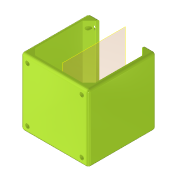
# Autodesk Inventor part: 55_spiralxy_slidemount_MGN9_Nema17_Body
Saved by Autodesk Inventor 2022 (Build 260153000, 153)
## iProperties
Created: 2019-07-01
Part Number: 55_spiralxy_slidemount_MGN9_Nema17_Body
Material: Generic
Document SubType Name: Modeling
Designer: diederichbenedict
Density: 1 g/cm^3
Appearance: IPHT_Grün
Author: diederichbenedict
Autodesk Inventor part; units mm, degrees
ref_plane "YZ Plane" through (0, 0, 0) normal (1, 0, 0) x (0, 1, 0)
ref_plane "XZ Plane" through (0, 0, 0) normal (0, 1, 0) x (-1, 0, 0)
ref_plane "XY Plane" through (0, 0, 0) normal (0, 0, 1) x (1, 0, 0)
sketch "Sketch1" plane through (0, 0, 0) normal (0, 0, 1) x (1, 0, 0)
  line L0 (-24.9, 24.9) -> (24.9, 24.9)
  line L1 (24.9, 24.9) -> (24.9, -24.9)
  line L2 (24.9, -24.9) -> (-24.9, -24.9)
  line L3 (-24.9, -24.9) -> (-24.9, 24.9)
  line L4 (-24.9, 24.9) -> (24.9, -24.9) construction
  line L5 (24.9, 24.9) -> (-24.9, -24.9) construction
  line L6 (17.05, 17.05) -> (-17.05, 17.05)
  line L7 (-17.05, 17.05) -> (-17.05, -17.05)
  line L8 (-17.05, -17.05) -> (17.05, -17.05)
  line L9 (17.05, -17.05) -> (17.05, 17.05)
  point P0 (0, 0)
  dimension "d0" = 49.8
  dimension "d1" = 49.8
  dimension "d2" = 7.85
  constraints: 20 end point, 4 parallel, 2 midpoint, 2 perpendicular, 1 horizontal, 3 other
  measures "d0" distance of L1.end L2.end
  measures "d1" distance of L0.end L1.end
  measures "d2" distance between parallel lines of L0 L6
extrude "Extrusion1" add sketch "Sketch1" along normal blind 7.7 contours L0 L1 L2 L3 | L9 L8 L7 L6
sketch "Sketch2" plane through (0, 0, 7.7) normal (0, 0, 1) x (1, 0, 0)
  line L0 (24.9, 24.9) -> (-24.9, 24.9) projected
  line L1 (-24.9, 24.9) -> (-24.9, -24.9) projected
  line L2 (-24.9, -24.9) -> (24.9, -24.9) projected
  line L3 (24.9, -24.9) -> (24.9, 24.9) projected
  line L4 (17.05, -17.05) -> (24.9, -17.05)
  line L5 (24.9, -17.05) -> (24.9, -24.9)
  line L6 (24.9, -24.9) -> (17.05, -24.9)
  line L7 (17.05, -24.9) -> (17.05, -17.05)
  line L8 (17.05, 17.05) -> (-17.05, 17.05) projected
  line L9 (24.9, 24.9) -> (17.05, 24.9)
  line L10 (17.05, 24.9) -> (17.05, 17.05)
  line L11 (17.05, 17.05) -> (24.9, 17.05)
  line L12 (24.9, 17.05) -> (24.9, 24.9)
  line L13 (-24.9, -24.9) -> (-17.05, -24.9)
  line L14 (-17.05, -24.9) -> (-17.05, -17.05)
  line L15 (-17.05, -17.05) -> (-24.9, -17.05)
  line L16 (-24.9, -17.05) -> (-24.9, -24.9)
  line L17 (-24.9, 24.9) -> (-17.05, 24.9)
  line L18 (-17.05, 24.9) -> (-17.05, 17.05)
  line L19 (-17.05, 17.05) -> (-24.9, 17.05)
  line L20 (-24.9, 17.05) -> (-24.9, 24.9)
  point P0 (0, 0)
  constraints: 32 end point, 8 parallel, 4 horizontal, 4 perpendicular
extrude "Extrusion2" add sketch "Sketch2" along normal blind 34.4
sketch "Sketch3" plane through (0, 0, 0) normal (0, 0, -1) x (-1, 0, 0)
  line L0 (24.9, -24.9) -> (24.9, 24.9) construction
  line L1 (24.9, 24.9) -> (-24.9, 24.9) construction
  line L2 (-24.9, -24.9) -> (24.9, -24.9) construction
  line L3 (-24.9, 24.9) -> (-24.9, -24.9) construction
  point P0 (20, 20)
  point P1 (20, -20)
  point P2 (-20, -20)
  point P3 (-20, 20)
  dimension "d_1" = 4.9
  dimension "d96" = 4.9
  dimension "d97" = 4.9
  dimension "d98" = 4.9
  dimension "d99" = 4.9
  dimension "d100" = 4.9
  dimension "d101" = 4.9
  dimension "d102" = 4.9
  measures "d_1" distance from line of L1 point (20, 20)
  measures "d96" distance from line of point (20, 20) L0
  measures "d97" distance from line of point (20, -20) L0
  measures "d98" distance from line of point (20, -20) L2
  measures "d99" distance from line of point (-20, -20) L2
  measures "d100" distance from line of point (-20, -20) L3
  measures "d101" distance from line of point (-20, 20) L3
  measures "d102" distance from line of point (-20, 20) L1
hole "Hole1" at (-20, 20, 0) at (-20, -20, 0) at (20, -20, 0) at (20, 20, 0) direction (0, 0, 1) diameter 2.8 end through all counterbore diameter 5.5 counterbore depth 3.1
fillet "Fillet1" radius 2 8 edges at (24.9, 24.9, 21.05) (24.9, -24.9, 21.05) (-24.9, -24.9, 21.05) (-24.9, 24.9, 21.05) (-24.9, 0, 0) (0, -24.9, 0) (24.9, 0, 0) (0, 24.9, 0)
sketch "Sketch9" plane through (0, 0, 42.1) normal (0, 0, 1) x (1, 0, 0)
  arc A0 (19.486, 18.6978) -> (18.6978, 19.486) centre (20, 20) ccw projected
  arc A1 (18.6978, -19.486) -> (19.486, -18.6978) centre (20, -20) ccw projected
  arc A2 (-19.486, -18.6978) -> (-18.6978, -19.486) centre (-20, -20) ccw projected
  arc A3 (-18.6978, 19.486) -> (-19.486, 18.6978) centre (-20, 20) ccw projected
hole "Hole2" at (20, 20, 42.1) at (-20, 20, 42.1) at (20, -20, 42.1) at (-20, -20, 42.1) direction (0, 0, -1) diameter 2.8 depth 12
sketch "Sketch15" plane through (0, 0, 0) normal (0, 0, -1) x (-1, 0, 0)
  circle A0 centre (-20, 20) radius 2.75 construction
  circle A1 centre (20, -20) radius 2.75 construction
  circle A2 centre (20, 20) radius 2.75 construction
  circle A3 centre (-20, -20) radius 2.75 construction
  line L0 (-22.9, 22.9) -> (22.9, 22.9) construction
  line L1 (-22.9, -22.9) -> (-22.9, 22.9) construction
  line L2 (22.9, -22.9) -> (-22.9, -22.9) construction
  line L3 (22.9, 22.9) -> (22.9, -22.9) construction
  line L4 (17.05, 21.1338) -> (-17.05, 21.1338) construction
  point P0 (0, 0)
  point P1 (-20.8, -14.5)
  point P2 (-14.5, -20.8)
  point P3 (14.5, -20.8)
  point P4 (20.8, -14.5)
  point P5 (20.8, 14.5)
  point P6 (14.5, 20.8)
  point P7 (-14.5, 20.8)
  point P8 (-20.8, 14.5)
hole "Hole8" [suppressed]
ref_plane "Arbeitsebene3" through (0, -17.05, 7.7) normal (1, 0, 0) x (0, 0, -1)
sketch "Skizze19" plane through (-22.9, -24.9, 42.1) normal (0, -1, 0) x (1, 0, 0)
  circle A0 centre (22.9, -17.2) radius 11.5 projected
  circle A1 centre (38.4, -1.7) radius 1.5 projected
  circle A2 centre (7.4, -1.7) radius 1.5 projected
  circle A3 centre (7.4, -32.7) radius 1.5 projected
  circle A4 centre (38.4, -32.7) radius 1.5 projected
  point P0 (22.9, -42.1)
hole "Bohrung9" at (-15.5, -24.9, 40.4) at (15.5, -24.9, 40.4) at (15.5, -24.9, 9.4) at (-15.5, -24.9, 9.4) direction (0, 1, 0) diameter 3 end through all
sketch "Skizze20" plane through (0, 0, 42.1) normal (0, 0, 1) x (1, 0, 0)
  line L0 (24.9, 22.9) -> (24.9, -22.9) projected
  arc A0 (22.9, -24.9) -> (24.9, -22.9) centre (22.9, -22.9) ccw projected
  line L1 (22.9, -24.9) -> (-22.9, -24.9) projected
  arc A1 (-24.9, -22.9) -> (-22.9, -24.9) centre (-22.9, -22.9) ccw projected
  line L2 (-24.9, -22.9) -> (-24.9, 22.9) projected
  arc A2 (-22.9, 24.9) -> (-24.9, 22.9) centre (-22.9, 22.9) ccw projected
  line L3 (-22.9, 24.9) -> (22.9, 24.9) projected
  arc A3 (24.9, 22.9) -> (22.9, 24.9) centre (22.9, 22.9) ccw projected
  circle A4 centre (-20, 20) radius 1.6 projected
  circle A5 centre (20, -20) radius 1.6 projected
  circle A6 centre (20, 20) radius 1.6 projected
  circle A7 centre (-20, -20) radius 1.6 projected
  arc A8 (21.65, 12.3091) -> (21.65, 16.6909) centre (20.8, 14.5) ccw projected
  line L4 (21.65, 17.05) -> (21.65, 16.6909) projected
  line L5 (21.65, 17.05) -> (17.05, 17.05) projected
  line L6 (17.05, 17.05) -> (17.05, 21.65) projected
  line L7 (17.05, 21.65) -> (16.6909, 21.65) projected
  arc A9 (16.6909, 21.65) -> (12.3091, 21.65) centre (14.5, 20.8) ccw projected
  line L8 (12.3091, 21.65) -> (-12.3091, 21.65) projected
  arc A10 (-12.3091, 21.65) -> (-16.6909, 21.65) centre (-14.5, 20.8) ccw projected
  line L9 (-16.6909, 21.65) -> (-17.05, 21.65) projected
  line L10 (-17.05, 21.65) -> (-17.05, 17.05) projected
  line L11 (-17.05, 17.05) -> (-21.65, 17.05) projected
  line L12 (-21.65, 16.6909) -> (-21.65, 17.05) projected
  arc A11 (-21.65, 16.6909) -> (-21.65, 12.3091) centre (-20.8, 14.5) ccw projected
  line L13 (-21.65, -12.3091) -> (-21.65, 12.3091) projected
  arc A12 (-21.65, -12.3091) -> (-21.65, -16.6909) centre (-20.8, -14.5) ccw projected
  line L14 (-21.65, -17.05) -> (-21.65, -16.6909) projected
  line L15 (-21.65, -17.05) -> (-17.05, -17.05) projected
  line L16 (-17.05, -17.05) -> (-17.05, -21.65) projected
  line L17 (-17.05, -21.65) -> (-16.6909, -21.65) projected
  arc A13 (-16.6909, -21.65) -> (-12.3091, -21.65) centre (-14.5, -20.8) ccw projected
  line L18 (-12.3091, -21.65) -> (12.3091, -21.65) projected
  arc A14 (12.3091, -21.65) -> (16.6909, -21.65) centre (14.5, -20.8) ccw projected
  line L19 (16.6909, -21.65) -> (17.05, -21.65) projected
  line L20 (17.05, -21.65) -> (17.05, -17.05) projected
  line L21 (17.05, -17.05) -> (21.65, -17.05) projected
  line L22 (21.65, -16.6909) -> (21.65, -17.05) projected
  arc A15 (21.65, -16.6909) -> (21.65, -12.3091) centre (20.8, -14.5) ccw projected
  line L23 (21.65, 12.3091) -> (21.65, -12.3091) projected
  line L24 (-17.05, 17.05) -> (-17.05, -17.05) projected
  line L25 (-17.05, 17.05) -> (-17.05, -17.05)
  line L26 (-21.2838, 17.05) -> (-17.05, 17.05) projected
  line L27 (-17.05, 17.05) -> (17.05, 17.05)
  line L28 (17.05, 17.05) -> (17.05, -17.05)
  line L29 (17.05, -17.05) -> (-17.05, -17.05)
  line L30 (-17.05, -17.05) -> (-17.05, 17.05)
  point P0 (0, 0)
  point P1 (-17.05, -17.05)
  constraints: 10 end point, 2 parallel, 1 collinear, 1 horizontal, 1 perpendicular
extrude "Extrusion8" add sketch "Skizze20" along normal blind 8 contours L0 A0 L1 A1 L2 A2 L3 A3 | L23 A15 L22 L21 L28 L5 L4 A8 | L27 L10 L9 A10 L8 A9 L7 L6 | L28 L29 L24 L27 | L24 L15 L14 A12 L13 A11 L12 L11 | L20 L19 A14 L18 A13 L17 L16 L29
fillet "Rundung2" radius 2 8 edges at (-24.3142, -24.3142, 50.1) (0, -24.9, 50.1) (24.3142, -24.3142, 50.1) (24.9, 0, 50.1) (24.3142, 24.3142, 50.1) (0, 24.9, 50.1) (-24.3142, 24.3142, 50.1) (-24.9, 0, 50.1)
sketch "Skizze18" plane through (-17.05, 24.9, 7.7) normal (0, 1, 0) x (1, 0, 0)
  line L0 (-4.1, -34.35) -> (-0.1, -38.35) projected
  line L1 (-0.1, -38.35) -> (2.9, -38.35) projected
  line L2 (-4.1, -31.35) -> (2.9, -38.35) projected
  line L3 (-4.1, -31.35) -> (-4.1, -34.35) projected
  line L4 (-4.1, -34.35) -> (-0.1, -38.35) projected
  line L5 (38.2, -31.35) -> (38.2, -3.05) projected
  line L6 (38.2, -3.05) -> (31.2, 3.95) projected
  line L7 (31.2, 3.95) -> (2.9, 3.95) projected
  line L8 (2.9, 3.95) -> (-4.1, -3.05) projected
  line L9 (-4.1, -3.05) -> (-4.1, -31.35) projected
  line L10 (-4.1, -31.35) -> (2.9, -38.35) projected
  line L11 (2.9, -38.35) -> (31.2, -38.35) projected
  line L12 (31.2, -38.35) -> (38.2, -31.35) projected
  circle A0 centre (17.05, -17.2) radius 2.5 projected
  circle A1 centre (1.55, -1.7) radius 1.5 projected
  circle A2 centre (1.55, -32.7) radius 1.5 projected
  circle A3 centre (32.55, -32.7) radius 1.5 projected
  circle A4 centre (32.55, -1.7) radius 1.5 projected
  circle A5 centre (17.05, -17.2) radius 4.6 projected
  line L13 (-4.1, -31.35) -> (-4.1, -3.05) projected
  line L14 (2.9, -38.35) -> (-4.1, -31.35) projected
  line L15 (31.2, -38.35) -> (2.9, -38.35) projected
  line L16 (38.2, -31.35) -> (31.2, -38.35) projected
  line L17 (38.2, -3.05) -> (38.2, -31.35) projected
  line L18 (31.2, 3.95) -> (38.2, -3.05) projected
  line L19 (2.9, 3.95) -> (31.2, 3.95) projected
  line L20 (-4.1, -3.05) -> (2.9, 3.95) projected
  line L21 (-0.1042, 3.95) -> (34.2, 3.95)
  line L22 (38.2, -0.05) -> (38.2, -34.35)
  line L23 (34.2, -38.35) -> (-0.1042, -38.35)
  line L24 (-4.1042, -34.35) -> (-4.1042, -0.05)
  line L25 (-4.1042, -0.05) -> (-0.1042, 3.95)
  line L26 (-4.1042, -34.35) -> (-0.1042, -38.35)
  line L27 (34.2, -38.35) -> (38.2, -34.35)
  line L28 (38.2, -0.05) -> (34.2, 3.95)
  line L29 (-0.5184, 4.95) -> (-5.1042, 0.3642)
  line L30 (-5.1042, 0.3642) -> (-5.1042, -34.7642)
  line L31 (-5.1042, -34.7642) -> (-0.5184, -39.35)
  line L32 (-0.5184, -39.35) -> (34.6142, -39.35)
  line L33 (34.6142, -39.35) -> (39.2, -34.7642)
  line L34 (39.2, -34.7642) -> (39.2, 0.3642)
  line L35 (39.2, 0.3642) -> (34.6142, 4.95)
  line L36 (34.6142, 4.95) -> (-0.5184, 4.95)
  point P0 (17.05, 7.7)
  point P1 (-4.1042, 3.95)
  point P2 (38.2, -38.35)
  point P3 (38.2, 3.95)
  point P4 (-4.1042, -38.35)
  dimension "d126" = 4
  dimension "d127" = 4
  dimension "d128" = 4
  dimension "d129" = 4
  dimension "d130" = 4
  dimension "d131" = 4
  dimension "d132" = 4
  dimension "d133" = 4
  dimension "d134" = 1
  constraints: 32 end point, 8 point on line, 4 parallel, 2 perpendicular, 1 horizontal, 7 other
  measures "d126" distance of L24.end point (-4.104, 3.95)
  measures "d127" distance of L21.start point (-4.104, 3.95)
  measures "d128" distance of L24.start point (-4.104, -38.35)
  measures "d129" distance of L23.end point (-4.104, -38.35)
  measures "d130" distance of L23.start point (38.2, -38.35)
  measures "d131" distance of L22.end point (38.2, -38.35)
  measures "d132" distance of L22.start point (38.2, 3.95)
  measures "d133" distance of L21.end point (38.2, 3.95)
  measures "d134" distance between parallel lines of L25 L29
extrude "Extrusion7" cut sketch "Skizze18" against normal blind 41.8 contours L3 L2 L1 L0 | L0 L23 L26 L24 L25 L21 L8 L9 L3 | L9 L8 L7 L6 L5 L12 L11 L2 | L12 L22 L27 L23 | L21 L28 L22 L6 | A0 | A1 | A2 | A3 | A4 | A5 | L36 L35 L34 L33 L32 L31 L30 L29
sketch "Skizze23" plane through (-22.9, 24.9, 2) normal (0, 1, 0) x (1, 0, 0)
  circle A0 centre (22.9, -22.9) radius 2.5 projected
  line L0 (15.4, -1.0242) -> (30.4, -1.0242)
  line L1 (30.4, -1.0242) -> (30.4, 5.0242)
  line L2 (30.4, 5.0242) -> (15.4, 5.0242)
  line L3 (15.4, 5.0242) -> (15.4, -1.0242)
  line L4 (15.4, -1.0242) -> (30.4, 5.0242) construction
  line L5 (30.4, -1.0242) -> (15.4, 5.0242) construction
  line L6 (5.85, 2) -> (5.85, -0.75) projected
  line L7 (40.15, 2) -> (45.65, 2) projected
  line L8 (39.95, 2) -> (39.95, -0.75) projected
  line L9 (5.85, 2) -> (39.95, 2)
  line L10 (39.95, 2) -> (39.95, -2.8792)
  line L11 (39.95, -2.8792) -> (5.85, -2.8792)
  line L12 (5.85, -2.8792) -> (5.85, 2)
  point P0 (22.9, 2)
  point P1 (15.4, 2)
  point P2 (5.85, -0.75)
  point P3 (30.4, 2)
  dimension "d156" = 15
  constraints: 20 end point, 4 parallel, 2 horizontal, 2 midpoint, 2 perpendicular, 1 point on line
  measures "d156" distance of L2.end L1.end
extrude "Extrusion10" cut sketch "Skizze23" against normal blind 42 contours L3 L9 L1 L0 | L0 L1 L9 L8 L10 L11 L12 L6 L3 | L3 L2 L1 L9
equation "\"d1\" = d0"
equation "\"d96\" = d_1"
equation "\"d97\" = d_1"
equation "\"d98\" = d_1"
equation "\"d99\" = d_1"
equation "\"d100\" = d_1"
equation "\"d101\" = d_1"
equation "\"d102\" = d_1"
body "Solid1"
